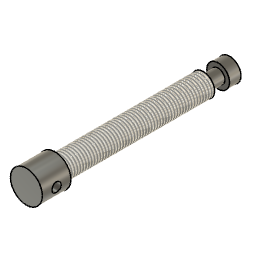
screw v1 (Autodesk Fusion 360 design; units mm, degrees)
Autodesk Fusion 360 part; units mm, degrees
sketch "Sketch1" plane through (0, 0, 0) normal (0, 1, 0) x (1, 0, 0)
  circle A0 centre (0, 0) radius 10
  circle A1 centre (0, 0) radius 6
  dimension "d1" = 20
  dimension "d2" = 12
  constraint coincident A0.centre A1.centre
  measures "d1" diameter of A0
  measures "d2" diameter of A1
extrude "Extrude1" add sketch "Sketch1" along normal blind 10 contours A0 | A1
extrude "Extrude3" add sketch "Sketch1" against normal blind 13 contours A1
extrude "Extrude4" add sketch "Sketch1" against normal blind 130 from surface at -13 contours A0 | A1
sketch "Sketch2" plane through (0, -143, 0) normal (0, -1, 0) x (1, 0, 0)
  circle A0 centre (0, 0) radius 10
  circle A1 centre (0, 0) radius 14
  dimension "d12" = 28
  constraint concentric A0 A1
  measures "d12" diameter of A1
extrude "Extrude5" add sketch "Sketch2" along normal blind 25 contours A0 | A1
thread "Thread1" "ISO Metric profile 20.0 M20x2.5 6g" major diameter 19.7905 minor diameter 16.938 pitch 2.5 angle 60 resizes the face on face at (9.9503, -56.3333, 0.9957)
sketch "Sketch3" plane through (0, 0, 0) normal (1, 0, 0) x (0, 1, 0)
  circle A0 centre (-155.5, 0) radius 4
  line L0 (-143, 14) -> (-143, -14)
  dimension "d15" = 8
  dimension "d20" = 12.5
  measures "d15" diameter of A0
  measures "d20" distance of A0.centre L0
extrude "Extrude6" cut sketch "Sketch3" along normal up to surface and the other way blind 14 end surface at (13.9826, -151.3333, 0.6978)
